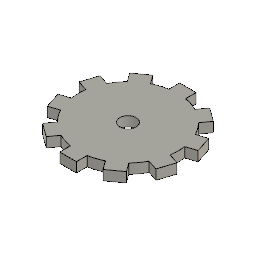
Flywheel idea v2 (Autodesk Fusion 360 design; units mm, degrees)
Autodesk Fusion 360 part; units mm, degrees
sketch "wheel" plane through (0, 0, 0) normal (0, 0, 1) x (1, 0, 0)
  circle A0 centre (0, 0) radius 19.05
  line L0 (-3.1964, 18.7799) -> (-3.1964, 22.86)
  line L1 (-3.1964, 22.86) -> (3.1964, 22.86)
  line L2 (3.1964, 22.86) -> (3.1964, 18.7799)
  line L3 (-13.6245, 13.3144) -> (-16.0227, 16.6153)
  line L4 (-16.0227, 16.6153) -> (-10.8508, 20.3729)
  line L5 (-10.8508, 20.3729) -> (-8.4526, 17.0721)
  line L6 (-18.8485, 2.7633) -> (-22.7289, 4.0241)
  line L7 (-22.7289, 4.0241) -> (-20.7534, 10.1041)
  line L8 (-20.7534, 10.1041) -> (-16.873, 8.8433)
  line L9 (-16.873, -8.8433) -> (-20.7534, -10.1041)
  line L10 (-20.7534, -10.1041) -> (-22.7289, -4.0241)
  line L11 (-22.7289, -4.0241) -> (-18.8485, -2.7633)
  line L12 (-8.4526, -17.0721) -> (-10.8508, -20.373)
  line L13 (-10.8508, -20.373) -> (-16.0227, -16.6153)
  line L14 (-16.0227, -16.6153) -> (-13.6245, -13.3145)
  line L15 (3.1964, -18.7799) -> (3.1964, -22.86)
  line L16 (3.1964, -22.86) -> (-3.1964, -22.86)
  line L17 (-3.1964, -22.86) -> (-3.1964, -18.7799)
  line L18 (13.6245, -13.3144) -> (16.0227, -16.6153)
  line L19 (16.0227, -16.6153) -> (10.8508, -20.3729)
  line L20 (10.8508, -20.3729) -> (8.4526, -17.0721)
  line L21 (18.8485, -2.7633) -> (22.7289, -4.0241)
  line L22 (22.7289, -4.0241) -> (20.7534, -10.1041)
  line L23 (20.7534, -10.1041) -> (16.873, -8.8433)
  line L24 (16.873, 8.8433) -> (20.7534, 10.1041)
  line L25 (20.7534, 10.1041) -> (22.7289, 4.0241)
  line L26 (22.7289, 4.0241) -> (18.8485, 2.7633)
  line L27 (8.4526, 17.0721) -> (10.8508, 20.373)
  line L28 (10.8508, 20.373) -> (16.0227, 16.6153)
  line L29 (16.0227, 16.6153) -> (13.6245, 13.3145)
  dimension "d1" = 38.1
  dimension "d2" = 6.3929
  dimension "d3" = 4.0801
  dimension "d5" = 360
  constraint coincident A0.centre origin
  constraint coincident A0 L0.start
  constraint vertical L0
  constraint perpendicular L0 L1
  constraint coincident A0 L2.end
  constraint perpendicular L1 L2
  constraint equal L0 L2
  measures "d1" diameter of A0
  measures "d2" distance of L0.end L1.end
  measures "d3" distance of L1.end L2.end
extrude "Extrude1" add sketch "wheel" along normal blind 3.81
sketch "hole punch" plane through (0, 0, 3.81) normal (0, 0, 1) x (-1, 0, 0)
  arc A0 (-8.4526, -17.0721) -> (-3.1964, -18.7799) centre (0, 0) ccw
  line L0 (-3.1964, -18.7799) -> (-3.1964, -22.86)
  line L1 (-3.1964, -22.86) -> (3.1964, -22.86)
  line L2 (3.1964, -22.86) -> (3.1964, -18.7799)
  arc A1 (3.1964, -18.7799) -> (8.4526, -17.0721) centre (0, 0) ccw
  line L3 (8.4526, -17.0721) -> (10.8508, -20.3729)
  line L4 (10.8508, -20.3729) -> (16.0227, -16.6153)
  line L5 (16.0227, -16.6153) -> (13.6245, -13.3144)
  arc A2 (13.6245, -13.3144) -> (16.873, -8.8433) centre (0, 0) ccw
  line L6 (16.873, -8.8433) -> (20.7534, -10.1041)
  line L7 (20.7534, -10.1041) -> (22.7289, -4.0241)
  line L8 (22.7289, -4.0241) -> (18.8485, -2.7633)
  arc A3 (18.8485, -2.7633) -> (18.8485, 2.7633) centre (0, 0) ccw
  line L9 (18.8485, 2.7633) -> (22.7289, 4.0241)
  line L10 (22.7289, 4.0241) -> (20.7534, 10.1041)
  line L11 (20.7534, 10.1041) -> (16.873, 8.8433)
  arc A4 (16.873, 8.8433) -> (13.6245, 13.3145) centre (0, 0) ccw
  line L12 (13.6245, 13.3145) -> (16.0227, 16.6153)
  line L13 (16.0227, 16.6153) -> (10.8508, 20.373)
  line L14 (10.8508, 20.373) -> (8.4526, 17.0721)
  arc A5 (8.4526, 17.0721) -> (3.1964, 18.7799) centre (0, 0) ccw
  line L15 (3.1964, 18.7799) -> (3.1964, 22.86)
  line L16 (3.1964, 22.86) -> (-3.1964, 22.86)
  line L17 (-3.1964, 22.86) -> (-3.1964, 18.7799)
  arc A6 (-3.1964, 18.7799) -> (-8.4526, 17.0721) centre (0, 0) ccw
  line L18 (-8.4526, 17.0721) -> (-10.8508, 20.3729)
  line L19 (-10.8508, 20.3729) -> (-16.0227, 16.6153)
  line L20 (-16.0227, 16.6153) -> (-13.6245, 13.3144)
  arc A7 (-13.6245, 13.3144) -> (-16.873, 8.8433) centre (0, 0) ccw
  line L21 (-16.873, 8.8433) -> (-20.7534, 10.1041)
  line L22 (-20.7534, 10.1041) -> (-22.7289, 4.0241)
  line L23 (-22.7289, 4.0241) -> (-18.8485, 2.7633)
  arc A8 (-18.8485, 2.7633) -> (-18.8485, -2.7633) centre (0, 0) ccw
  line L24 (-18.8485, -2.7633) -> (-22.7289, -4.0241)
  line L25 (-22.7289, -4.0241) -> (-20.7534, -10.1041)
  line L26 (-20.7534, -10.1041) -> (-16.873, -8.8433)
  arc A9 (-16.873, -8.8433) -> (-13.6245, -13.3145) centre (0, 0) ccw
  line L27 (-13.6245, -13.3145) -> (-16.0227, -16.6153)
  line L28 (-16.0227, -16.6153) -> (-10.8508, -20.373)
  line L29 (-10.8508, -20.373) -> (-8.4526, -17.0721)
  circle A10 centre (0, 0) radius 19.05
  line L30 (0.0528, -19.0499) -> (0.0528, 19.0499)
  line L31 (19.05, 0) -> (-19.05, 0)
  constraint coincident A0.centre A1.centre
  constraint coincident A10 L30.start
  constraint coincident A10 L30.end
  constraint vertical L30
  constraint midpoint A3 L31.start
  constraint midpoint A8 L31.end
hole "Hole1" at (0, 0, 3.81) direction (0, 0, -1) diameter 6.2 depth 6.2 tip angle 118
